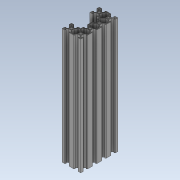
# Autodesk Inventor part: perfil2
Saved by Autodesk Inventor 2022 (Build 260153000, 153)
## iProperties
Created: 2022-03-21
Part Number: perfil2
Material: Generic
Document SubType Name: Modeling
Designer: ferna
Density: 1 g/cm^3
Appearance: Chrome - Polished Black
Mass: 186.971 g
Surface Area: 2100.81 cm^2
Volume: 186.971 cm^3
Author: ferna
Autodesk Inventor part; units mm, degrees
ref_plane "YZ Plane" through (0, 0, 0) normal (1, 0, 0) x (0, 1, 0)
ref_plane "XZ Plane" through (0, 0, 0) normal (0, 1, 0) x (-1, 0, 0)
ref_plane "XY Plane" through (0, 0, 0) normal (0, 0, 1) x (1, 0, 0)
sketch "Sketch1" plane through (0, 0, 0) normal (0, 1, 0) x (-1, 0, 0)
  line L0 (20, 0) -> (20, -5.2)
  line L1 (18.7, -6.5) -> (18.2, -6.5)
  line L2 (18.2, -6.5) -> (18.7, -6.5)
  line L3 (18.7, -6.5) -> (20, -5.2)
  line L4 (20, -6.5) -> (20.5385, -6.5) construction
  line L5 (20, 0) -> (20, -5.2)
  line L6 (20, -14.8) -> (20, -20)
  line L7 (20, 0) -> (14.8, 0)
  line L8 (13.5, -1.3) -> (13.5, -1.8)
  line L9 (13.5, -1.8) -> (13.5, -1.3)
  line L10 (13.5, -1.3) -> (14.8, 0)
  line L11 (13.5, -1.8) -> (15.5, -1.8)
  line L12 (18.2, -6.5) -> (18.2, -4.5)
  line L13 (18.2, -4.5) -> (16.4, -4.5)
  line L14 (15.5, -1.8) -> (15.5, -3.6)
  line L15 (18.2, -18.2) -> (20, -20)
  circle A0 centre (10, -10) radius 2.3
  line L16 (12.95, -6.15) -> (7.05, -6.15)
  line L17 (6.15, -7.05) -> (6.15, -12.95)
  line L18 (7.05, -13.85) -> (12.95, -13.85)
  line L19 (13.85, -12.95) -> (13.85, -7.05)
  line L20 (13.85, -6.15) -> (8.3737, -11.6263) construction
  line L21 (6.15, -6.15) -> (13.85, -13.85) construction
  line L22 (15.5, -1.8) -> (15.5, -3.6)
  line L23 (18.2, -4.5) -> (16.4, -4.5)
  line L24 (16.4, -4.5) -> (13.85, -7.05)
  line L25 (15.5, -3.6) -> (12.95, -6.15)
  line L26 (0, 0) -> (13.5, 0)
  line L27 (14.8, 0) -> (20, 0)
  line L28 (20, -20) -> (20, -14.8)
  line L29 (18.7, -13.5) -> (18.2, -13.5)
  line L30 (18.2, -13.5) -> (18.7, -13.5)
  line L31 (18.7, -13.5) -> (20, -14.8)
  line L32 (20, -13.5) -> (20.5385, -13.5) construction
  line L33 (20, -20) -> (20, -14.8)
  line L34 (20, -20) -> (14.8, -20)
  line L35 (13.5, -18.7) -> (13.5, -18.2)
  line L36 (13.5, -18.2) -> (13.5, -18.7)
  line L37 (13.5, -18.7) -> (14.8, -20)
  line L38 (13.5, -18.2) -> (15.5, -18.2)
  line L39 (18.2, -13.5) -> (18.2, -15.5)
  line L40 (18.2, -15.5) -> (16.4, -15.5)
  line L41 (15.5, -18.2) -> (15.5, -16.4)
  line L42 (15.5, -18.2) -> (15.5, -16.4)
  line L43 (18.2, -15.5) -> (16.4, -15.5)
  line L44 (16.4, -15.5) -> (13.85, -12.95)
  line L45 (15.5, -16.4) -> (12.95, -13.85)
  line L46 (14.8, -20) -> (20, -20)
  line L47 (15.2, -10) -> (15.5, -10)
  line L48 (6.15, -13.85) -> (6.5, -13.5)
  line L49 (4.5, -16.4) -> (7.05, -13.85)
  line L50 (3.6, -15.5) -> (6.15, -12.95)
  line L51 (0, -13.5) -> (-0.5385, -13.5) construction
  line L52 (4.5, -18.2) -> (4.5, -16.4)
  line L53 (4.5, -18.2) -> (4.5, -16.4)
  line L54 (0, -20) -> (5.2, -20)
  line L55 (3.65, -20) -> (0, -20)
  line L56 (6.5, -18.2) -> (4.5, -18.2)
  line L57 (6.5, -18.7) -> (6.5, -18.2)
  line L58 (6.5, -18.2) -> (6.5, -18.7)
  line L59 (6.5, -18.7) -> (5.2, -20)
  line L60 (6.15, -6.15) -> (6.5, -6.5)
  line L61 (3.6, -4.5) -> (6.15, -7.05)
  line L62 (4.5, -1.8) -> (4.5, -3.6)
  line L63 (4.5, -1.8) -> (4.5, -3.6)
  line L64 (0, 0) -> (5.2, 0)
  line L65 (5.2, 0) -> (0, 0)
  line L66 (0, -6.5) -> (-0.5385, -6.5) construction
  line L67 (4.5, -3.6) -> (7.05, -6.15)
  line L68 (6.5, -1.8) -> (4.5, -1.8)
  line L69 (6.5, -1.3) -> (6.5, -1.8)
  line L70 (6.5, -1.3) -> (5.2, 0)
  line L71 (6.5, -1.8) -> (6.5, -1.3)
  line L72 (-20, 0) -> (-20, -5.2)
  line L73 (-18.7, -6.5) -> (-18.2, -6.5)
  line L74 (-18.2, -6.5) -> (-18.7, -6.5)
  line L75 (-18.7, -6.5) -> (-20, -5.2)
  line L76 (-20, -6.5) -> (-20.5385, -6.5) construction
  line L77 (-20, 0) -> (-20, -5.2)
  line L78 (-20, -14.8) -> (-20, -20)
  line L79 (-20, 0) -> (-14.8, 0)
  line L80 (-13.5, -1.3) -> (-13.5, -1.8)
  line L81 (-13.5, -1.8) -> (-13.5, -1.3)
  line L82 (-13.5, -1.3) -> (-14.8, 0)
  line L83 (-13.5, -1.8) -> (-15.5, -1.8)
  line L84 (-18.2, -6.5) -> (-18.2, -4.5)
  line L85 (-18.2, -4.5) -> (-16.4, -4.5)
  line L86 (-15.5, -1.8) -> (-15.5, -3.6)
  line L87 (-19.55, -19.55) -> (-20, -20)
  circle A1 centre (-10, -10) radius 2.3
  line L88 (-12.95, -6.15) -> (-7.05, -6.15)
  line L89 (-6.15, -7.05) -> (-6.15, -12.95)
  line L90 (-7.05, -13.85) -> (-12.95, -13.85)
  line L91 (-13.85, -12.95) -> (-13.85, -7.05)
  line L92 (-13.85, -6.15) -> (-8.3737, -11.6263) construction
  line L93 (-6.15, -6.15) -> (-13.85, -13.85) construction
  line L94 (-15.5, -1.8) -> (-15.5, -3.6)
  line L95 (-18.2, -4.5) -> (-16.4, -4.5)
  line L96 (-16.4, -4.5) -> (-13.85, -7.05)
  line L97 (-15.5, -3.6) -> (-12.95, -6.15)
  line L98 (0, 0) -> (-13.5, 0)
  line L99 (-14.8, 0) -> (-20, 0)
  line L100 (-18.7, -13.5) -> (-18.2, -13.5)
  line L101 (-18.2, -13.5) -> (-18.7, -13.5)
  line L102 (-18.7, -13.5) -> (-20, -14.8)
  line L103 (-15.5, -16.4) -> (-12.95, -13.85)
  line L104 (-18.2, -15.5) -> (-16.4, -15.5)
  line L105 (-16.4, -15.5) -> (-13.85, -12.95)
  line L106 (-18.2, -13.5) -> (-18.2, -15.5)
  line L107 (-20, -13.5) -> (-20.5385, -13.5) construction
  line L108 (-18.2, -15.5) -> (-16.4, -15.5)
  line L109 (-20, -20) -> (-20, -14.8)
  line L110 (-20, -20) -> (-20, -14.8)
  line L111 (-15.2, -10) -> (-15.5, -10)
  line L112 (-6.15, -13.85) -> (-6.5, -13.5)
  line L113 (-3.6, -15.5) -> (-6.15, -12.95)
  line L114 (0, -13.5) -> (0.5385, -13.5) construction
  line L115 (-4.5, -16.4) -> (-7.05, -13.85)
  line L116 (-6.15, -6.15) -> (-6.5, -6.5)
  line L117 (-6.5, -1.3) -> (-6.5, -1.8)
  line L118 (-6.5, -1.8) -> (-6.5, -1.3)
  line L119 (-4.5, -3.6) -> (-7.05, -6.15)
  line L120 (-3.6, -4.5) -> (-6.15, -7.05)
  line L121 (-6.5, -1.8) -> (-4.5, -1.8)
  line L122 (-6.5, -1.3) -> (-5.2, 0)
  line L123 (-4.5, -1.8) -> (-4.5, -3.6)
  line L124 (-4.5, -1.8) -> (-4.5, -3.6)
  line L125 (-5.2, 0) -> (0, 0)
  line L126 (0, 0) -> (-5.2, 0)
  line L127 (0, -6.5) -> (0.5385, -6.5) construction
  line L128 (3.6, -4.5) -> (3.15, -4.05)
  line L129 (1.8, -1.8) -> (3.15, -1.8)
  line L130 (3.15, -1.8) -> (3.15, -4.05)
  line L131 (1.8, -1.8) -> (-3.4, -1.8)
  line L132 (-3.6, -4.5) -> (-3.15, -4.05)
  line L133 (-3.15, -4.05) -> (-3.15, -1.8)
  line L134 (6.5, -18.7) -> (6.5, -18.2)
  line L135 (6.5, -18.2) -> (6.5, -18.7)
  line L136 (6.5, -18.2) -> (4.5, -18.2)
  line L137 (6.5, -18.7) -> (5.2, -20)
  line L138 (4.5, -18.2) -> (4.5, -16.4)
  line L139 (4.5, -18.2) -> (4.5, -16.4)
  line L140 (3.65, -20) -> (0, -20)
  line L141 (0, -20) -> (3.65, -20)
  line L142 (1.8, -18.2) -> (3.15, -18.2)
  line L143 (3.15, -18.2) -> (3.15, -15.95)
  line L144 (1.8, -18.2) -> (-0.9, -18.2)
  line L145 (-3.15, -15.95) -> (-3.6, -15.5)
  line L146 (3.6, -15.5) -> (3.15, -15.95)
  line L147 (20, -20) -> (14.8, -20)
  line L148 (3.65, -20) -> (0, -20)
  line L149 (0, -26.5) -> (-0.5385, -26.5) construction
  line L150 (0, -33.5) -> (-0.5385, -33.5) construction
  line L151 (-20, -33.5) -> (-20.5385, -33.5) construction
  line L152 (-18.7, -33.5) -> (-20, -34.8)
  line L153 (-18.2, -35.5) -> (-16.4, -35.5)
  line L154 (-18.2, -35.5) -> (-16.4, -35.5)
  line L155 (-18.7, -33.5) -> (-18.2, -33.5)
  line L156 (-18.2, -33.5) -> (-18.7, -33.5)
  line L157 (-18.2, -33.5) -> (-18.2, -35.5)
  line L158 (-16.4, -35.5) -> (-13.85, -32.95)
  line L159 (-20, -40) -> (-20, -34.8)
  line L160 (-20, -40) -> (-20, -34.8)
  line L161 (-15.5, -36.4) -> (-12.95, -33.85)
  line L162 (-12.95, -33.85) -> (-7.05, -33.85)
  line L163 (-13.85, -33.85) -> (-8.3737, -28.3737) construction
  circle A2 centre (-10, -30) radius 2.3
  line L164 (-6.15, -33.85) -> (-13.85, -26.15) construction
  line L165 (-6.15, -32.95) -> (-6.15, -27.05)
  line L166 (-7.05, -26.15) -> (-12.95, -26.15)
  line L167 (-15.2, -30) -> (-15.5, -30)
  line L168 (-13.85, -27.05) -> (-13.85, -32.95)
  line L169 (-16.4, -24.5) -> (-13.85, -27.05)
  line L170 (-15.5, -23.6) -> (-12.95, -26.15)
  line L171 (-20, -25.2) -> (-20, -20)
  line L172 (-19.55, -20.45) -> (-20, -20)
  line L173 (-18.2, -24.5) -> (-16.4, -24.5)
  line L174 (-18.2, -24.5) -> (-16.4, -24.5)
  line L175 (-18.2, -26.5) -> (-18.2, -24.5)
  line L176 (-18.7, -26.5) -> (-18.2, -26.5)
  line L177 (-18.2, -26.5) -> (-18.7, -26.5)
  line L178 (-18.7, -26.5) -> (-20, -25.2)
  line L179 (-15.5, -23.15) -> (-15.5, -23.6)
  line L180 (-20, -20) -> (-20, -25.2)
  line L181 (-20, -20) -> (-20, -25.2)
  line L182 (-20, -26.5) -> (-20.5385, -26.5) construction
  line L183 (-6.15, -26.15) -> (-6.5, -26.5)
  line L184 (-4.5, -23.6) -> (-7.05, -26.15)
  line L185 (-4.5, -25.4) -> (-6.15, -27.05)
  line L186 (0, -26.5) -> (0.5385, -26.5) construction
  line L187 (-6.15, -33.85) -> (-6.5, -33.5)
  line L188 (0, -33.5) -> (0.5385, -33.5) construction
  line L189 (-3.15, -15.95) -> (-0.9, -18.2)
  line L190 (-3.15, -15.95) -> (0.032, -15.95) construction
  line L191 (-4.5, -16.4) -> (-2.7, -18.2)
  line L192 (-4.5, -16.4) -> (-1.9544, -16.4) construction
  line L193 (-2.7, -18.2) -> (-1.8, -19.1)
  line L194 (-1.8, -19.1) -> (-1.8, -23.15)
  line L195 (-1.8, -23.15) -> (-4.05, -23.15)
  line L196 (-4.05, -23.15) -> (-4.5, -23.6)
  line L197 (-1.8, -23.15) -> (-1.8, -23.4)
  line L198 (-1.8, -24.5) -> (-3.6, -24.5)
  line L199 (-3.6, -24.5) -> (-4.5, -25.4)
  line L200 (-1.8, -24.5) -> (-1.8, -26.5)
  line L201 (-1.8, -26.5) -> (-1.3, -26.5)
  line L202 (0, -24.95) -> (0, -20)
  line L203 (-1.3, -26.5) -> (0, -25.2)
  line L204 (0, -25.2) -> (0, -24.95)
  line L205 (-15.5, -16.4) -> (-15.95, -16.85)
  line L206 (-18.2, -15.5) -> (-18.2, -15.95)
  line L207 (-18.2, -16.4) -> (-18.2, -16.85)
  line L208 (-18.2, -16.85) -> (-15.95, -16.85)
  line L209 (-19.1, -20) -> (-20, -20)
  line L210 (-20, -20) -> (-19.1, -20)
  line L211 (-18.2, -23.15) -> (-15.95, -23.15)
  line L212 (-15.95, -23.15) -> (-15.5, -23.6)
  line L213 (-18.2, -16.85) -> (-18.2, -23.15)
  line L214 (-18.2, -35.5) -> (-18.2, -36.85)
  line L215 (-18.2, -36.85) -> (-15.95, -36.85)
  line L216 (-15.95, -36.85) -> (-15.5, -36.4)
  line L217 (-18.2, -36.85) -> (-18.2, -40)
  line L218 (-18.2, -40) -> (-13.5, -40)
  line L219 (-5.25, -33.85) -> (-6.15, -32.95)
  line L220 (-6.15, -34.75) -> (-7.05, -33.85)
  line L221 (-3.6, -35.5) -> (-5.25, -33.85)
  line L222 (-4.05, -36.85) -> (-6.15, -34.75)
  line L223 (-3.6, -35.5) -> (-1.8, -35.5)
  line L224 (-1.8, -35.5) -> (-1.8, -33.5)
  line L225 (-1.8, -33.5) -> (-1.3, -33.5)
  line L226 (-1.3, -33.5) -> (0, -34.8)
  line L227 (0, -34.8) -> (0, -36.85)
  line L228 (-4.05, -36.85) -> (-1.8, -36.85)
  line L229 (-1.8, -36.85) -> (-1.8, -40)
  line L230 (0, -36.85) -> (0, -40)
  line L231 (20, -80) -> (20, -74.8)
  line L232 (18.7, -73.5) -> (18.2, -73.5)
  line L233 (18.2, -73.5) -> (18.7, -73.5)
  line L234 (18.7, -73.5) -> (20, -74.8)
  line L235 (20, -73.5) -> (20.5385, -73.5) construction
  line L236 (20, -80) -> (20, -74.8)
  line L237 (20, -65.2) -> (20, -60)
  line L238 (20, -80) -> (14.8, -80)
  line L239 (13.5, -78.7) -> (13.5, -78.2)
  line L240 (13.5, -78.2) -> (13.5, -78.7)
  line L241 (13.5, -78.7) -> (14.8, -80)
  line L242 (13.5, -78.2) -> (15.5, -78.2)
  line L243 (18.2, -73.5) -> (18.2, -75.5)
  line L244 (18.2, -75.5) -> (16.4, -75.5)
  line L245 (15.5, -78.2) -> (15.5, -76.4)
  line L246 (18.2, -61.8) -> (20, -60)
  circle A3 centre (10, -70) radius 2.3
  line L247 (12.95, -73.85) -> (7.05, -73.85)
  line L248 (6.15, -72.95) -> (6.15, -67.05)
  line L249 (7.05, -66.15) -> (12.95, -66.15)
  line L250 (13.85, -67.05) -> (13.85, -72.95)
  line L251 (13.85, -73.85) -> (8.3737, -68.3737) construction
  line L252 (6.15, -73.85) -> (13.85, -66.15) construction
  line L253 (15.5, -78.2) -> (15.5, -76.4)
  line L254 (18.2, -75.5) -> (16.4, -75.5)
  line L255 (16.4, -75.5) -> (13.85, -72.95)
  line L256 (15.5, -76.4) -> (12.95, -73.85)
  line L257 (0, -80) -> (13.5, -80)
  line L258 (14.8, -80) -> (20, -80)
  line L259 (18.7, -66.5) -> (18.2, -66.5)
  line L260 (18.2, -66.5) -> (18.7, -66.5)
  line L261 (18.7, -66.5) -> (20, -65.2)
  line L262 (15.5, -63.6) -> (12.95, -66.15)
  line L263 (18.2, -64.5) -> (16.4, -64.5)
  line L264 (16.4, -64.5) -> (13.85, -67.05)
  line L265 (18.2, -66.5) -> (18.2, -64.5)
  line L266 (20, -66.5) -> (20.5385, -66.5) construction
  line L267 (18.2, -64.5) -> (16.4, -64.5)
  line L268 (20, -60) -> (20, -65.2)
  line L269 (15.5, -61.8) -> (15.5, -63.6)
  line L270 (15.5, -61.8) -> (15.5, -63.6)
  line L271 (20, -60) -> (20, -65.2)
  line L272 (20, -60) -> (14.8, -60)
  line L273 (14.8, -60) -> (20, -60)
  line L274 (13.5, -61.8) -> (15.5, -61.8)
  line L275 (13.5, -61.3) -> (13.5, -61.8)
  line L276 (13.5, -61.8) -> (13.5, -61.3)
  line L277 (13.5, -61.3) -> (14.8, -60)
  line L278 (15.2, -70) -> (15.5, -70)
  line L279 (6.15, -66.15) -> (6.5, -66.5)
  line L280 (3.6, -64.5) -> (6.15, -67.05)
  line L281 (4.5, -61.8) -> (4.5, -63.6)
  line L282 (4.5, -61.8) -> (4.5, -63.6)
  line L283 (0, -60) -> (5.2, -60)
  line L284 (3.65, -60) -> (0, -60)
  line L285 (0, -66.5) -> (-0.5385, -66.5) construction
  line L286 (4.5, -63.6) -> (7.05, -66.15)
  line L287 (6.5, -61.8) -> (4.5, -61.8)
  line L288 (6.5, -61.3) -> (6.5, -61.8)
  line L289 (6.5, -61.3) -> (5.2, -60)
  line L290 (6.5, -61.8) -> (6.5, -61.3)
  line L291 (6.15, -73.85) -> (6.5, -73.5)
  line L292 (6.5, -78.7) -> (6.5, -78.2)
  line L293 (6.5, -78.2) -> (6.5, -78.7)
  line L294 (4.5, -76.4) -> (7.05, -73.85)
  line L295 (3.6, -75.5) -> (6.15, -72.95)
  line L296 (6.5, -78.2) -> (4.5, -78.2)
  line L297 (6.5, -78.7) -> (5.2, -80)
  line L298 (4.5, -78.2) -> (4.5, -76.4)
  line L299 (4.5, -78.2) -> (4.5, -76.4)
  line L300 (5.2, -80) -> (0, -80)
  line L301 (0, -80) -> (5.2, -80)
  line L302 (0, -73.5) -> (-0.5385, -73.5) construction
  line L303 (-20, -73.5) -> (-20.5385, -73.5) construction
  line L304 (-18.7, -73.5) -> (-20, -74.8)
  line L305 (-18.2, -75.5) -> (-16.4, -75.5)
  line L306 (-18.2, -75.5) -> (-16.4, -75.5)
  line L307 (-18.7, -73.5) -> (-18.2, -73.5)
  line L308 (-18.2, -73.5) -> (-18.7, -73.5)
  line L309 (-18.2, -73.5) -> (-18.2, -75.5)
  line L310 (-16.4, -75.5) -> (-13.85, -72.95)
  line L311 (-15.5, -78.2) -> (-15.5, -76.4)
  line L312 (-15.5, -78.2) -> (-15.5, -76.4)
  line L313 (-20, -80) -> (-20, -74.8)
  line L314 (-20, -80) -> (-20, -74.8)
  line L315 (-20, -80) -> (-14.8, -80)
  line L316 (-14.8, -80) -> (-20, -80)
  line L317 (-13.5, -78.2) -> (-15.5, -78.2)
  line L318 (-13.5, -78.7) -> (-13.5, -78.2)
  line L319 (-13.5, -78.2) -> (-13.5, -78.7)
  line L320 (-13.5, -78.7) -> (-14.8, -80)
  line L321 (-15.5, -76.4) -> (-12.95, -73.85)
  line L322 (-12.95, -73.85) -> (-7.05, -73.85)
  line L323 (-13.85, -73.85) -> (-8.3737, -68.3737) construction
  circle A4 centre (-10, -70) radius 2.3
  line L324 (-6.15, -73.85) -> (-13.85, -66.15) construction
  line L325 (-6.15, -72.95) -> (-6.15, -67.05)
  line L326 (-7.05, -66.15) -> (-12.95, -66.15)
  line L327 (-15.2, -70) -> (-15.5, -70)
  line L328 (-13.85, -67.05) -> (-13.85, -72.95)
  line L329 (-16.4, -64.5) -> (-13.85, -67.05)
  line L330 (-15.5, -63.6) -> (-12.95, -66.15)
  line L331 (-20, -65.2) -> (-20, -60)
  line L332 (-19.55, -60.45) -> (-20, -60)
  line L333 (-18.2, -64.5) -> (-16.4, -64.5)
  line L334 (-18.2, -64.5) -> (-16.4, -64.5)
  line L335 (-18.2, -66.5) -> (-18.2, -64.5)
  line L336 (-18.7, -66.5) -> (-18.2, -66.5)
  line L337 (-18.2, -66.5) -> (-18.7, -66.5)
  line L338 (-18.7, -66.5) -> (-20, -65.2)
  line L339 (-20, -60) -> (-20, -65.2)
  line L340 (-20, -60) -> (-20, -65.2)
  line L341 (-20, -66.5) -> (-20.5385, -66.5) construction
  line L342 (-6.15, -66.15) -> (-6.5, -66.5)
  line L343 (-4.5, -63.6) -> (-7.05, -66.15)
  line L344 (-3.6, -64.5) -> (-6.15, -67.05)
  line L345 (0, -66.5) -> (0.5385, -66.5) construction
  line L346 (-6.5, -78.7) -> (-6.5, -78.2)
  line L347 (-6.5, -78.2) -> (-4.5, -78.2)
  line L348 (-6.5, -78.7) -> (-5.2, -80)
  line L349 (-6.5, -78.2) -> (-6.5, -78.7)
  line L350 (0, -80) -> (-13.5, -80)
  line L351 (-6.15, -73.85) -> (-6.5, -73.5)
  line L352 (-4.5, -78.2) -> (-4.5, -76.4)
  line L353 (-4.5, -78.2) -> (-4.5, -76.4)
  line L354 (-4.5, -76.4) -> (-7.05, -73.85)
  line L355 (-3.6, -75.5) -> (-6.15, -72.95)
  line L356 (-5.2, -80) -> (0, -80)
  line L357 (0, -80) -> (-5.2, -80)
  line L358 (0, -73.5) -> (0.5385, -73.5) construction
  line L359 (3.6, -75.5) -> (3.15, -75.95)
  line L360 (1.8, -78.2) -> (3.15, -78.2)
  line L361 (3.15, -78.2) -> (3.15, -75.95)
  line L362 (1.8, -78.2) -> (-3.4, -78.2)
  line L363 (-3.6, -75.5) -> (-3.15, -75.95)
  line L364 (-3.15, -75.95) -> (-3.15, -78.2)
  line L365 (1.8, -61.8) -> (-0.9, -61.8)
  line L366 (1.8, -61.8) -> (3.15, -61.8)
  line L367 (6.5, -61.3) -> (6.5, -61.8)
  line L368 (6.5, -61.8) -> (6.5, -61.3)
  line L369 (6.5, -61.8) -> (4.5, -61.8)
  line L370 (4.5, -61.8) -> (4.5, -63.6)
  line L371 (6.5, -61.3) -> (5.2, -60)
  line L372 (3.65, -60) -> (0, -60)
  line L373 (0, -60) -> (3.65, -60)
  line L374 (4.5, -61.8) -> (4.5, -63.6)
  line L375 (3.15, -61.8) -> (3.15, -64.05)
  line L376 (-3.15, -64.05) -> (-3.6, -64.5)
  line L377 (3.6, -64.5) -> (3.15, -64.05)
  line L378 (20, -60) -> (14.8, -60)
  line L379 (3.65, -60) -> (0, -60)
  line L380 (0, -53.5) -> (-0.5385, -53.5) construction
  line L381 (0, -53.5) -> (0.5385, -53.5) construction
  line L382 (0, -46.5) -> (0.5385, -46.5) construction
  line L383 (0, -46.5) -> (-0.5385, -46.5) construction
  line L384 (-6.15, -46.15) -> (-6.5, -46.5)
  line L385 (-20, -46.5) -> (-20.5385, -46.5) construction
  line L386 (-18.7, -46.5) -> (-20, -45.2)
  line L387 (-18.2, -44.5) -> (-16.4, -44.5)
  line L388 (-18.2, -44.5) -> (-16.4, -44.5)
  line L389 (-18.7, -46.5) -> (-18.2, -46.5)
  line L390 (-18.2, -46.5) -> (-18.7, -46.5)
  line L391 (-18.2, -46.5) -> (-18.2, -44.5)
  line L392 (-20, -40) -> (-20, -45.2)
  line L393 (-20, -40) -> (-20, -45.2)
  line L394 (-16.4, -55.5) -> (-13.85, -52.95)
  line L395 (-15.5, -56.4) -> (-12.95, -53.85)
  line L396 (-20, -54.8) -> (-20, -60)
  line L397 (-15.5, -56.85) -> (-15.5, -56.4)
  line L398 (-18.2, -55.5) -> (-16.4, -55.5)
  line L399 (-18.2, -55.5) -> (-16.4, -55.5)
  line L400 (-19.55, -59.55) -> (-20, -60)
  line L401 (-20, -60) -> (-20, -54.8)
  line L402 (-20, -60) -> (-20, -54.8)
  line L403 (-18.2, -53.5) -> (-18.2, -55.5)
  line L404 (-18.7, -53.5) -> (-18.2, -53.5)
  line L405 (-18.2, -53.5) -> (-18.7, -53.5)
  line L406 (-18.7, -53.5) -> (-20, -54.8)
  line L407 (-20, -53.5) -> (-20.5385, -53.5) construction
  line L408 (-6.15, -53.85) -> (-6.5, -53.5)
  line L409 (-4.5, -56.4) -> (-7.05, -53.85)
  line L410 (-4.5, -54.6) -> (-6.15, -52.95)
  line L411 (-16.4, -44.5) -> (-13.85, -47.05)
  line L412 (-15.5, -43.6) -> (-12.95, -46.15)
  line L413 (-12.95, -46.15) -> (-7.05, -46.15)
  line L414 (-13.85, -46.15) -> (-8.3737, -51.6263) construction
  circle A5 centre (-10, -50) radius 2.3
  line L415 (-6.15, -46.15) -> (-13.85, -53.85) construction
  line L416 (-6.15, -47.05) -> (-6.15, -52.95)
  line L417 (-7.05, -53.85) -> (-12.95, -53.85)
  line L418 (-15.2, -50) -> (-15.5, -50)
  line L419 (-13.85, -52.95) -> (-13.85, -47.05)
  line L420 (-3.15, -64.05) -> (-0.9, -61.8)
  line L421 (-3.15, -64.05) -> (0.032, -64.05) construction
  line L422 (-4.5, -63.6) -> (-2.7, -61.8)
  line L423 (-4.5, -63.6) -> (-1.9544, -63.6) construction
  line L424 (-2.7, -61.8) -> (-1.8, -60.9)
  line L425 (-1.8, -60.9) -> (-1.8, -56.85)
  line L426 (-1.8, -56.85) -> (-4.05, -56.85)
  line L427 (-4.05, -56.85) -> (-4.5, -56.4)
  line L428 (-1.8, -56.85) -> (-1.8, -56.6)
  line L429 (-1.8, -55.5) -> (-3.6, -55.5)
  line L430 (-3.6, -55.5) -> (-4.5, -54.6)
  line L431 (-1.8, -55.5) -> (-1.8, -53.5)
  line L432 (-1.8, -53.5) -> (-1.3, -53.5)
  line L433 (0, -55.05) -> (0, -60)
  line L434 (-1.3, -53.5) -> (0, -54.8)
  line L435 (0, -54.8) -> (0, -55.05)
  line L436 (-15.5, -63.6) -> (-15.95, -63.15)
  line L437 (-18.2, -64.5) -> (-18.2, -64.05)
  line L438 (-18.2, -63.6) -> (-18.2, -63.15)
  line L439 (-18.2, -63.15) -> (-15.95, -63.15)
  line L440 (-19.1, -60) -> (-20, -60)
  line L441 (-20, -60) -> (-19.1, -60)
  line L442 (-18.2, -56.85) -> (-15.95, -56.85)
  line L443 (-15.95, -56.85) -> (-15.5, -56.4)
  line L444 (-18.2, -63.15) -> (-18.2, -56.85)
  line L445 (-18.2, -44.5) -> (-18.2, -43.15)
  line L446 (-18.2, -43.15) -> (-15.95, -43.15)
  line L447 (-15.95, -43.15) -> (-15.5, -43.6)
  line L448 (-18.2, -43.15) -> (-18.2, -40)
  line L449 (-5.25, -46.15) -> (-6.15, -47.05)
  line L450 (-6.15, -45.25) -> (-7.05, -46.15)
  line L451 (-3.6, -44.5) -> (-5.25, -46.15)
  line L452 (-4.05, -43.15) -> (-6.15, -45.25)
  line L453 (-3.6, -44.5) -> (-1.8, -44.5)
  line L454 (-1.8, -44.5) -> (-1.8, -46.5)
  line L455 (-1.8, -46.5) -> (-1.3, -46.5)
  line L456 (-1.3, -46.5) -> (0, -45.2)
  line L457 (0, -45.2) -> (0, -43.15)
  line L458 (-4.05, -43.15) -> (-1.8, -43.15)
  line L459 (-1.8, -43.15) -> (-1.8, -40)
  line L460 (0, -43.15) -> (0, -40)
  point P0 (13.5, -20)
  point P1 (6.5, -20)
  point P2 (8.3737, -8.3737)
  point P3 (1.8, -4.5)
  point P4 (6.5, 0)
  point P5 (-18.2, -18.2)
  point P6 (-15.5, -18.2)
  point P7 (-13.5, -20)
  point P8 (-4.5, -18.2)
  point P9 (-6.5, -20)
  point P10 (-8.3737, -8.3737)
  point P11 (-6.5, 0)
  point P12 (-1.8, -4.5)
  point P13 (-1.8, -1.8)
  point P14 (6.5, -20)
  point P15 (-6.5, -20)
  point P16 (-3.4, -18.2)
  point P17 (-3.15, -18.2)
  point P18 (13.5, -40)
  point P19 (1.8, -21.8)
  point P20 (1.8, -38.2)
  point P21 (-15.5, -38.2)
  point P22 (-13.5, -38.7)
  point P23 (-18.2, -21.8)
  point P24 (-15.5, -21.8)
  point P25 (-6.5, -40)
  point P26 (-1.8, -38.2)
  point P27 (-8.3737, -31.6263)
  point P28 (13.5, -60)
  point P29 (6.5, -60)
  point P30 (8.3737, -71.6263)
  point P31 (6.5, -80)
  point P32 (1.8, -75.5)
  point P33 (-18.2, -61.8)
  point P34 (-15.5, -61.8)
  point P35 (-13.5, -60)
  point P36 (-4.5, -61.8)
  point P37 (-6.5, -60)
  point P38 (-6.5, -80)
  point P39 (-1.8, -78.2)
  point P40 (-1.8, -75.5)
  point P41 (-8.3737, -71.6263)
  point P42 (-3.4, -61.8)
  point P43 (-6.5, -60)
  point P44 (-3.15, -61.8)
  point P45 (6.5, -60)
  point P46 (-13.5, -41.3)
  point P47 (-15.5, -41.8)
  point P48 (-15.5, -58.2)
  point P49 (-18.2, -58.2)
  point P50 (-8.3737, -48.3737)
  point P51 (1.8, -58.2)
  point P52 (-1.8, -41.8)
  point P53 (1.8, -41.8)
  point P54 (-5.2, 0)
  dimension "d12" = 4.6
  dimension "d2" = 6.5
  dimension "d3" = 1.8
  dimension "d4" = 0.5
  dimension "d5" = 45
  dimension "d7" = 1.8
  dimension "d8" = 2
  dimension "d9" = 2
  dimension "d13" = 7.7
  dimension "d14" = 7.7
  dimension "d15" = 1.8
  dimension "d16" = 1.8
  dimension "d17" = 45
  dimension "d18" = 45
  dimension "d19" = 4.05
  dimension "d20" = 1.35
  dimension "d21" = 2
  dimension "d22" = 0.5
  dimension "d24" = 1.8
  dimension "d25" = 1.35
  dimension "d26" = 1.35
  dimension "d27" = 1.35
  dimension "d28" = 3.15
  dimension "d29" = 2
  dimension "d30" = 135
  dimension "d31" = 3.15
  constraints: 922 end point, 302 symmetric about line, 56 point on line, 24 perpendicular, 13 horizontal, 9 parallel, 9 vertical, 6 coincident, 6 midpoint, 2 collinear, 2 equal length, 18 other
  measures "d2" distance of L4.start L0.start
  measures "d3" distance of L4.start L1.end
  measures "d4" distance of L1.start L1.end
  measures "d5" angle of L4 L3
  measures "d7" distance of L26.end L8.end
  measures "d8" distance of L8.end L11.end
  measures "d9" distance of L1.end L12.end
  measures "d13" distance of L48.start L21.end
  measures "d14" distance of L48.start L21.start
  measures "d15" distance of L14.end L11.end
  measures "d16" distance of L13.end L12.end
  measures "d17" angle of L189 L190
  measures "d18" angle of L191 L192
  measures "d19" distance of L193.end L194.end
  measures "d20" distance between parallel lines of L143 L52
  measures "d21" distance of L198.start L200.end
  measures "d22" distance of L200.end L201.end
  measures "d24" distance between parallel lines of L200 L202
  measures "d25" distance between parallel lines of L123 L133
  measures "d26" distance of L104.start L207.end
  measures "d27" distance of L153.start L214.end
  measures "d28" distance of L214.end L217.end
  measures "d29" distance of L223.end L224.end
  measures "d30" angle of L225 L226
  measures "d31" distance of L228.end L229.end
extrude "Extrusion1" add sketch "Sketch1" along normal blind 250 contours L0 L3 L1 L12 L13 L24 L19 L44 L40 L39 L29 L31 L6 L34 L37 L35 L38 L41 L45 L18 L49 L52 L56 L57 L59 L54 L202 L204 L203 L201 L200 L198 L199 L185 L165 L219 L221 L223 L224 L225 L226 L227 L230 L460 L457 L456 L455 L454 L453 L451 L449 L416 L410 L430 L429 L431 L432 L434 L435 L433 L283 L289 L288 L287 L281 L286 L249 L262 L269 L274 L275 L277 L272 L237 L261 L259 L265 L263 L264 L250 L255 L244 L243 L232 L234 L231 L238 L241 L239 L242 L245 L256 L247 L294 L298 L296 L292 L297 L257 L350 L348 L346 L347 L352 L354 L322 L321 L311 L317 L318 L320 L315 L313 L304 L307 L309 L305 L310 L328 L329 L333 L335 L336 L338 L331 L396 L406 L404 L403 L398 L394 L419 L411 L387 L445 L446 L447 L412 L413 L450 L452 L458 L459 L229 L228 L222 L220 L162 L161 L216 L215 L214 L153 L158 L168 L169 L173 L175 L176 L178 L171 L78 L102 L100 L106 L104 L105 L91 L96 L85 L84 L73 L75 L72 L79 L82 L80 L83 L86 L97 L88 L119 L123 L121 L117 L122 L98 L26 L70 L69 L68 L62 L67 L16 L25 L14 L11 L8 L10 L7 | L214 L217 L448 L445 L391 L389 L386 L392 L159 L152 L155 L157
body "Solid1"
